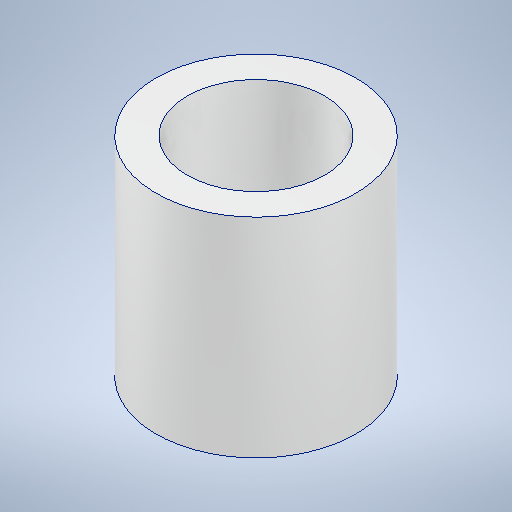
# Autodesk Inventor part: Spacers for Rollers
Saved by Autodesk Inventor 2025 (Build 290162000, 162)
## iProperties
Created: 2025-03-12
Part Number: Spacers for Rollers
Material: Aluminum 6061
Document SubType Name: Modeling
Designer: MAL16204
Mass: 0.597605 g
Surface Area: 4.0715 cm^2
Volume: 0.221335 cm^3
Density: 2.7 g/cm^3
Appearance: Aluminum - Flat
Manager: J. Wilburn
Title: Spacers for Rollers
Subject: Ender 3 Pro Assembly
Author: Richard Malstrom
Autodesk Inventor part; units mm, degrees
ref_plane "YZ Plane" through (0, 0, 0) normal (1, 0, 0) x (0, 1, 0)
ref_plane "XZ Plane" through (0, 0, 0) normal (0, 1, 0) x (-1, 0, 0)
ref_plane "XY Plane" through (0, 0, 0) normal (0, 0, 1) x (1, 0, 0)
sketch "Sketch1" plane through (0, 0, 0) normal (0, 1, 0) x (-1, 0, 0)
  circle A0 centre (0, 0) radius 4
  circle A1 centre (0, 0) radius 2.75
  dimension "d0" = 8
  dimension "d1" = 5.5
  constraints: 2 centre point, 2 coincident
  measures "d0" diameter of A0
  measures "d1" diameter of A1
extrude "Extrusion1" add sketch "Sketch1" along normal blind 8.35
body "Solid1"
